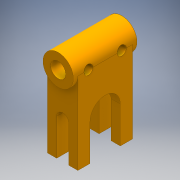
# Autodesk Inventor part: Forcella
Saved by Autodesk Inventor 2016 (Build 200138000, 138)
## iProperties
Created: 2016-09-10
Part Number: Forcella
Material: Generic
Document SubType Name: Modeling
Designer: Muhammad
Density: 1 g/cm^3
Appearance: Default
Author: Muhammad
Autodesk Inventor part; units mm, degrees
ref_plane "YZ Plane" through (0, 0, 0) normal (1, 0, 0) x (0, 1, 0)
ref_plane "XZ Plane" through (0, 0, 0) normal (0, 1, 0) x (-1, 0, 0)
ref_plane "XY Plane" through (0, 0, 0) normal (0, 0, 1) x (1, 0, 0)
sketch "Sketch1" plane through (0, 0, 0) normal (0, 1, 0) x (-1, 0, 0)
  circle A0 centre (0, 0) radius 5
  circle A1 centre (0, 0) radius 2.5
  constraints: 2 centre point, 2 coincident
extrude "Extrusion1" add sketch "Sketch1" along normal mid plane 21
sketch "Sketch2" plane through (0, 0, 0) normal (0, 1, 0) x (-1, 0, 0)
  circle A0 centre (0, 0) radius 5 construction
  line L0 (5, 0) -> (5, -27) construction
  line L1 (5, 0) -> (-5, 0)
  line L2 (-5, 0) -> (-5, -27)
  line L3 (-5, -27) -> (5, -27)
  line L4 (5, -27) -> (5, 0)
  dimension "d4" = 27
  constraints: 10 end point, 2 parallel, 2 vertical, 1 horizontal, 1 horizontal alignment, 1 perpendicular, 1 other
  measures "d4" distance of L0.start L0.end
extrude "Extrusion2" add sketch "Sketch2" along normal mid plane 18
sketch "Sketch3" plane through (0, 9, 0) normal (0, 1, 0) x (1, 0, 0)
  circle A0 centre (0, 0) radius 2.5
  constraints: 1 centre point, 1 coincident
extrude "Extrusion3" cut sketch "Sketch3" against normal blind 18
sketch "Sketch4" plane through (0, 9, 0) normal (0, 1, 0) x (1, 0, 0)
  line L0 (5, 0) -> (5, 27) projected
  arc A0 (-2, 15) -> (2, 15) centre (0, 15) ccw
  line L1 (2, 27) -> (2, 15)
  line L2 (-2, 27) -> (-2, 15)
  line L3 (2, 27) -> (-2, 27)
  line L4 (5, 27) -> (-5, 27) projected
  point P0 (0, 0)
  constraints: 6 end point, 2 point on circle, 2 tangent, 1 centre point, 1 collinear
extrude "Extrusion4" cut sketch "Sketch4" against normal through all
sketch "Sketch5" plane through (-5, -9, 0) normal (-1, 0, 0) x (0, 0, 1)
  line L0 (-27, 18) -> (-27, 14) construction
  line L1 (-27, 14) -> (-27, 4)
  line L2 (-27, 0) -> (-27, 18) projected
  line L3 (-27, 9) -> (-10, 9) construction
  arc A0 (-15, 4) -> (-15, 14) centre (-15, 9) ccw
  line L4 (-27, 14) -> (-15, 14)
  line L5 (-27, 4) -> (-15, 4)
  point P0 (0, 9)
  dimension "d16" = 10
  dimension "d17" = 17
  constraints: 10 end point, 2 point on circle, 2 point on line, 2 tangent, 1 centre point, 1 horizontal, 1 midpoint
  measures "d16" distance of L0.end L1.end
  measures "d17" distance of L3.start L3.end
extrude "Extrusion5" cut sketch "Sketch5" against normal through all
sketch "Sketch7" plane through (5, -9, 0) normal (1, 0, 0) x (0, 0, -1)
  line L0 (-5, -1.5) -> (5, -1.5) construction
  line L1 (0, -1.5) -> (0, 3.5) construction
  line L2 (0, 0) -> (0, 18) construction
  line L3 (5, 19.5) -> (-5, 19.5) construction
  line L4 (0, 19.5) -> (0, 14.5) construction
  circle A0 centre (0, 3.5) radius 1.5
  circle A1 centre (0, 14.5) radius 1.5
  point P0 (0, 9)
  dimension "d28" = 5
  dimension "d29" = 5
  dimension "d30" = 3
  dimension "d31" = 3
  constraints: 4 end point, 2 centre point, 2 coincident, 2 midpoint, 2 point on line
  measures "d28" distance of L1.start L1.end
  measures "d29" distance of L4.start L4.end
  measures "d30" diameter of A0
  measures "d31" diameter of A1
extrude "Extrusion7" cut sketch "Sketch7" against normal up to surface
body "Solid1"
